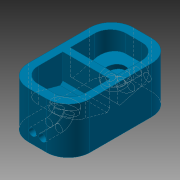
# Autodesk Inventor part: Line Tracker v3
Saved by Autodesk Inventor 2015 (Build 190159000, 159)
## iProperties
Created: 2015-04-19
Part Number: Line Tracker v3
Material: PLA Plastic
Document SubType Name: Modeling
Designer: Kyle
Density: 1 g/cm^3
Appearance: Carbon Fiber 1
Author: Kyle
Autodesk Inventor part; units mm, degrees
ref_plane "YZ Plane" through (0, 0, 0) normal (1, 0, 0) x (0, 1, 0)
ref_plane "XZ Plane" through (0, 0, 0) normal (0, 1, 0) x (-1, 0, 0)
ref_plane "XY Plane" through (0, 0, 0) normal (0, 0, 1) x (1, 0, 0)
sketch "Sketch1" plane through (0, 0, 0) normal (1, 0, 0) x (0, 1, 0)
  line L0 (0, 0) -> (0, 10.795)
  line L1 (0, 10.795) -> (9.525, 10.795)
  line L2 (9.525, 10.795) -> (9.525, 9.017)
  line L3 (9.525, 9.017) -> (5.8775, 9.017)
  line L4 (5.8775, 9.017) -> (3.81, 1.3008)
  line L5 (4.3488, 0.762) -> (9.525, 0.762)
  line L6 (9.525, 0.762) -> (9.525, 0)
  line L7 (0, 0) -> (9.525, 0) construction
  line L8 (3.81, 1.3008) -> (4.3488, 0.762)
  line L9 (0, 0) -> (0, -10.795)
  line L10 (0, -10.795) -> (9.525, -10.795)
  line L11 (9.525, -10.795) -> (9.525, -9.017)
  line L12 (9.525, -9.017) -> (5.8775, -9.017)
  line L13 (5.8775, -9.017) -> (3.81, -1.3008)
  line L14 (4.3488, -0.762) -> (9.525, -0.762)
  line L15 (9.525, -0.762) -> (9.525, 0)
  line L16 (3.81, -1.3008) -> (4.3488, -0.762)
  dimension "d0" = 10.795
  dimension "d1" = 105
  dimension "d8" = 0.762
  dimension "d33" = 3.81
  dimension "d34" = 9.525
  dimension "d35" = 0.762
  dimension "d36" = 1.778
  constraints: 34 end point, 7 symmetric about line, 4 perpendicular, 2 horizontal, 1 collinear, 1 vertical
  measures "d0" distance of L0.start L0.end
  measures "d1" angle of L4 L3
  measures "d8" distance of L5.end L6.end
  measures "d33" distance from line of L0 L4.end
  measures "d34" distance of L0.end L1.end
  measures "d35" distance of L4.end L5.start
  measures "d36" distance of L1.end L2.end
extrude "Extrusion1" add sketch "Sketch1" along normal mid plane 9.652
sketch "Sketch2" plane through (4.826, 0, 0) normal (1, 0, 0) x (0, 0, -1)
  line L0 (-10.795, 9.525) -> (10.795, 9.525)
  line L1 (10.795, 9.525) -> (10.795, 0)
  line L2 (10.795, 0) -> (-10.795, 0)
  line L3 (-10.795, 0) -> (-10.795, 9.525)
  point P0 (0, 0)
  constraints: 8 end point, 2 parallel, 1 coincident, 1 horizontal, 1 perpendicular
extrude "Extrusion2" add sketch "Sketch2" along normal blind 1.524
ref_plane "Work Plane1" through (0, 0, 0) normal (-1, 0, 0) x (0, 0, 1)
mirror "Mirror1" about plane through (0, 0, 0) normal (-1, 0, 0) of "Extrusion2"
ref_plane "Work Plane2" through (4.826, 5.8775, 0) normal (0, 0, 1) x (1, 0, 0)
sketch "Sketch3" plane through (-4.826, 3.81, -1.3008) normal (0, 0.9659258, 0.258819) x (1, 0, 0)
  circle A0 centre (4.826, 3.8534) radius 2.286
  line L0 (4.826, -2.2426) -> (4.826, 3.8534) construction
  line L1 (9.652, 0.9587) -> (0, 0.9587) construction
  dimension "d14" = 4.572
  dimension "d15" = 6.096
  constraints: 2 end point, 1 centre point, 1 perpendicular
  measures "d14" diameter of A0
  measures "d15" distance of L0.start L0.end
extrude "Extrusion3" cut sketch "Sketch3" against normal blind 1.016
mirror "Mirror2" about plane through (4.826, 5.8775, 0) normal (0, 0, 1) of "Extrusion3"
sketch "Sketch4" plane through (0, 3.826, 5.2859) normal (0, 0.9659258, -0.258819) x (1, 0, 0)
  line L0 (0, 0) -> (1.016, 0)
  circle A0 centre (1.016, 0) radius 0.762
  line L1 (0, 0) -> (0, -1.5045) construction
  line L2 (0, 0) -> (-1.016, 0)
  circle A1 centre (-1.016, 0) radius 0.762
  line L3 (-4.0349, -2.2244) -> (3.3383, -2.2244) construction
  point P0 (0, 6.096)
  dimension "d18" = 1.016
  dimension "d19" = 1.524
  constraints: 8 end point, 2 centre point, 2 coincident, 2 horizontal, 2 symmetric about line, 1 vertical, 1 other
  measures "d18" distance of L0.start L0.end
  measures "d19" diameter of A0
revolve "Revolution1" cut sketch "Sketch4" angle 75 about axis through (-4.0349, 4.4017, 7.4344) along (-1, 0, 0)
mirror "Mirror3" about plane through (4.826, 5.8775, 0) normal (0, 0, 1) of "Revolution1"
sketch "Sketch6" plane through (1.016, 2.1773, -7.4344) normal (0, 0, 1) x (1, 0, 0)
  circle A0 centre (0, 0) radius 0.762
  circle A1 centre (0, 0) radius 0.762 projected
  point P0 (-1.016, -2.1773)
  dimension "d37" = 1.524
  constraints: 1 centre point, 1 concentric
  measures "d37" diameter of A0
extrude "Extrusion5" cut sketch "Sketch6" against normal up to next
mirror "Mirror8" about plane through (0, 0, 0) normal (-1, 0, 0) of "Extrusion5"
mirror "Mirror9" about plane through (4.826, 5.8775, 0) normal (0, 0, 1) of "Extrusion5", "Mirror8"
fillet "Fillet4" radius 3.175 4 edges at (4.826, 7.7013, -9.017) (-4.826, 7.7013, -9.017) (4.826, 7.7013, 9.017) (-4.826, 7.7013, 9.017)
fillet "Fillet5" radius 4.445 4 edges at (6.35, 4.7625, 10.795) (6.35, 4.7625, -10.795) (-6.35, 4.7625, -10.795) (-6.35, 4.7625, 10.795)
equation "\"d0\" = 0.5 * Base_Length"
equation "\"d1\" = Sensor_Angle"
equation "\"d33\" = Base_Thickness"
equation "\"d34\" = Mount_Height"
equation "\"d14\" = LED_Base"
equation "\"d15\" = Hole_to_Center"
equation "\"d18\" = Wire_Spacing"
equation "\"d19\" = Wire_Diameter"
equation "\"d37\" = Wire_Diameter"
equation "\"Wire_Spacing\" = 1.016"
equation "\"Wire_Diameter\" = 1.524"
equation "\"LED_Base\" = 4.572"
equation "\"Mount_Space\" = 12.7"
equation "\"Mount_Clearance\" = 3.175"
equation "\"Mount_Height\" = Mount_Space - Mount_Clearance"
equation "\"Base_Length\" = 21.59"
equation "\"Base_Width\" = 12.7"
equation "\"Sensor_Angle\" = 105deg"
equation "\"Base_Thickness\" = 3.81"
equation "\"Hole_to_Center\" = 6.096"
body "Solid1"
